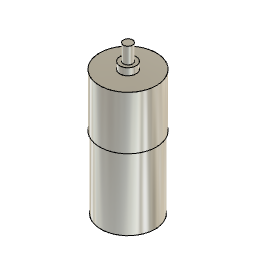
Line Spool (Autodesk Fusion 360 archive; units mm, degrees)
design "Motor"
Autodesk Fusion 360 part; units mm, degrees
sketch "Sketch1" plane through (0, 0, 0) normal (0, 0, 1) x (1, 0, 0) in component "Motor v2"
  circle A0 centre (0, 0) radius 12.25
  circle A1 centre (0, 0) radius 3.5
  circle A2 centre (0, 0) radius 2
  dimension "d1_2_1_1_1" = 24.5
  dimension "d8_1_1_1_1" = 7
  dimension "d9_1_1_1_1" = 4
  dimension "d478_1_1" = 0
  dimension "d479_1_1" = 0
  dimension "d480_1_1" = 0
  dimension "d481_1_1" = 0
  constraint coincident A0.centre A1.centre
  constraint concentric A0 A1
  constraint concentric A1 A2
  measures "d1_2_1_1_1" diameter of A0
  measures "d8_1_1_1_1" diameter of A1
  measures "d9_1_1_1_1" diameter of A2
ref_plane "WorkPlane1" through (0, 0, -23) normal (0, 0, 1) x (1, 0, 0) in component "Motor v2"
sketch "Sketch2" plane through (0, 0, -23) normal (0, 0, 1) x (1, 0, 0) in component "Motor v2"
  circle A0 centre (0, 0) radius 11.75
  dimension "d3_3_1_1" = 23.5
  constraint coincident A0.centre origin
  measures "d3_3_1_1" diameter of A0
extrude "Extrude1" add sketch "Sketch1" against normal blind 23 contours A0 | A1 | A2 in component "Motor v2"
extrude "Extrude2" add sketch "Sketch2" against normal blind 31 in component "Motor v2"
extrude "Extrude3" add sketch "Sketch1" along normal blind 3 contours A1 | A2 in component "Motor v2"
extrude "Extrude4" add sketch "Sketch1" along normal blind 10 contours A2 in component "Motor v2"
component "Motor v2" placed x (1, 0, 0) y (0, 1, 0) z (0, 0, 1) at (0, 0, 0)
equation "d1_2_1_1_1 = 23.5 mm + 1 mm"
